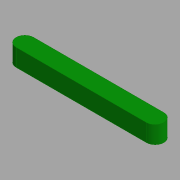
# Autodesk Inventor part: LED green
Saved by Autodesk Inventor 2014 SP2 (Build 180246200, 246)
## iProperties
Created: 2016-01-21
Part Number: LED green
Material: ABS plast
Document SubType Name: Modeling
Designer: Mervart
Mass: 0.0702602 g
Surface Area: 1.3885 cm^2
Volume: 0.0662832 cm^3
Density: 1.06 g/cm^3
Appearance: Hladká – bílá
LastSaveDate: 21.09.2010
Hmotnost: 0
Author: Mervart
Autodesk Inventor part; units mm, degrees
ref_plane "YZ Plane" through (0, 0, 0) normal (1, 0, 0) x (0, 1, 0)
ref_plane "XZ Plane" through (0, 0, 0) normal (0, 1, 0) x (-1, 0, 0)
ref_plane "XY Plane" through (0, 0, 0) normal (0, 0, 1) x (1, 0, 0)
sketch "Náčrt4" plane through (0, 0, 0) normal (0, 0, 1) x (1, 0, 0)
  line L0 (-23.962, 1.2647) -> (-8.962, 1.2647) construction
  line L1 (-8.962, -0.7353) -> (-23.962, -0.7353) construction
  line L2 (-41.962, 1.2647) -> (-26.962, 1.2647) construction
  line L3 (-26.962, -0.7353) -> (-41.962, -0.7353) construction
  line L4 (-59.962, 1.2647) -> (-44.962, 1.2647) construction
  line L5 (-44.962, -0.7353) -> (-59.962, -0.7353) construction
  line L6 (-59.962, 14.7647) -> (-0.822, 14.7647) construction
  arc A0 (-59.962, 14.7647) -> (-69.262, 5.4647) centre (-59.962, 5.4647) ccw construction
  line L7 (-69.262, -84.5353) -> (-69.262, 5.4647) construction
  arc A1 (-69.262, -84.5353) -> (-59.962, -93.8353) centre (-59.962, -84.5353) ccw construction
  line L8 (2.038, -93.8353) -> (-59.962, -93.8353) construction
  line L9 (2.038, -93.8353) -> (2.038, 0.4647) construction
  line L10 (2.038, 0.4647) -> (-0.822, 14.7647) construction
  line L11 (-60.962, -18.7353) -> (-60.962, -4.7353) construction
  line L12 (-59.462, -3.2353) -> (-45.462, -3.2353) construction
  line L13 (-43.962, -4.7353) -> (-43.962, -18.7353) construction
  line L14 (-45.462, -20.2353) -> (-59.462, -20.2353) construction
  circle A2 centre (-34.452, 10.9647) radius 0.3 construction
  circle A3 centre (-30.952, 7.4647) radius 0.3 construction
  circle A4 centre (-34.452, 3.9647) radius 0.3 construction
  circle A5 centre (-37.952, 7.4647) radius 0.3 construction
  circle A6 centre (-34.452, 7.4647) radius 0.3 construction
  circle A7 centre (-36.9269, 9.9395) radius 0.3 construction
  circle A8 centre (-36.9269, 4.9898) radius 0.3 construction
  circle A9 centre (-31.9771, 4.9898) radius 0.3 construction
  circle A10 centre (-31.9771, 9.9395) radius 0.3 construction
  line L15 (-59.962, 1.2647) -> (-44.962, 1.2647)
  line L16 (-44.962, -0.7353) -> (-59.962, -0.7353)
  line L17 (-29.7605, -84.0301) -> (-30.334, -84.8493) projected
  arc A11 (-30.334, -84.8493) -> (-38.5901, -84.8493) centre (-34.462, -90.7447) ccw projected
  line L18 (-38.5901, -84.8493) -> (-39.1636, -84.0301) projected
  arc A12 (-29.7605, -84.0301) -> (-39.1636, -84.0301) centre (-34.462, -90.7447) ccw projected
  circle A13 centre (-34.462, -90.7447) radius 0.9 projected
  line L19 (-31.9385, -86.548) -> (-32.512, -87.3672) projected
  arc A14 (-32.512, -87.3672) -> (-36.412, -87.3672) centre (-34.462, -90.7447) ccw projected
  line L20 (-36.412, -87.3672) -> (-36.9856, -86.548) projected
  arc A15 (-31.9385, -86.548) -> (-36.9856, -86.548) centre (-34.462, -90.7447) ccw projected
  arc A16 (-27.8677, -81.3269) -> (-41.0564, -81.3269) centre (-34.462, -90.7447) ccw projected
  line L21 (-27.8677, -81.3269) -> (-28.4412, -82.1461) projected
  arc A17 (-28.4412, -82.1461) -> (-40.4829, -82.1461) centre (-34.462, -90.7447) ccw projected
  line L22 (-40.4829, -82.1461) -> (-41.0564, -81.3269) projected
  line L23 (-24.962, -72.7353) -> (-24.962, -58.7353) projected
  arc A18 (-23.462, -57.2353) -> (-24.962, -58.7353) centre (-23.462, -58.7353) ccw projected
  line L24 (-23.462, -57.2353) -> (-9.462, -57.2353) projected
  arc A19 (-7.962, -58.7353) -> (-9.462, -57.2353) centre (-9.462, -58.7353) ccw projected
  line L25 (-7.962, -58.7353) -> (-7.962, -72.7353) projected
  arc A20 (-9.462, -74.2353) -> (-7.962, -72.7353) centre (-9.462, -72.7353) ccw projected
  line L26 (-9.462, -74.2353) -> (-23.462, -74.2353) projected
  arc A21 (-24.962, -72.7353) -> (-23.462, -74.2353) centre (-23.462, -72.7353) ccw projected
  line L27 (-42.962, -72.7353) -> (-42.962, -58.7353) projected
  arc A22 (-41.462, -57.2353) -> (-42.962, -58.7353) centre (-41.462, -58.7353) ccw projected
  line L28 (-41.462, -57.2353) -> (-27.462, -57.2353) projected
  arc A23 (-25.962, -58.7353) -> (-27.462, -57.2353) centre (-27.462, -58.7353) ccw projected
  line L29 (-25.962, -58.7353) -> (-25.962, -72.7353) projected
  arc A24 (-27.462, -74.2353) -> (-25.962, -72.7353) centre (-27.462, -72.7353) ccw projected
  line L30 (-27.462, -74.2353) -> (-41.462, -74.2353) projected
  arc A25 (-42.962, -72.7353) -> (-41.462, -74.2353) centre (-41.462, -72.7353) ccw projected
  line L31 (-60.962, -72.7353) -> (-60.962, -58.7353) projected
  arc A26 (-59.462, -57.2353) -> (-60.962, -58.7353) centre (-59.462, -58.7353) ccw projected
  line L32 (-59.462, -57.2353) -> (-45.462, -57.2353) projected
  arc A27 (-43.962, -58.7353) -> (-45.462, -57.2353) centre (-45.462, -58.7353) ccw projected
  line L33 (-43.962, -58.7353) -> (-43.962, -72.7353) projected
  arc A28 (-45.462, -74.2353) -> (-43.962, -72.7353) centre (-45.462, -72.7353) ccw projected
  line L34 (-45.462, -74.2353) -> (-59.462, -74.2353) projected
  arc A29 (-60.962, -72.7353) -> (-59.462, -74.2353) centre (-59.462, -72.7353) ccw projected
  line L35 (-24.962, -54.7353) -> (-24.962, -40.7353) projected
  arc A30 (-23.462, -39.2353) -> (-24.962, -40.7353) centre (-23.462, -40.7353) ccw projected
  line L36 (-23.462, -39.2353) -> (-9.462, -39.2353) projected
  arc A31 (-7.962, -40.7353) -> (-9.462, -39.2353) centre (-9.462, -40.7353) ccw projected
  line L37 (-7.962, -40.7353) -> (-7.962, -54.7353) projected
  arc A32 (-9.462, -56.2353) -> (-7.962, -54.7353) centre (-9.462, -54.7353) ccw projected
  line L38 (-9.462, -56.2353) -> (-23.462, -56.2353) projected
  arc A33 (-24.962, -54.7353) -> (-23.462, -56.2353) centre (-23.462, -54.7353) ccw projected
  line L39 (-42.962, -54.7353) -> (-42.962, -40.7353) projected
  arc A34 (-41.462, -39.2353) -> (-42.962, -40.7353) centre (-41.462, -40.7353) ccw projected
  line L40 (-41.462, -39.2353) -> (-27.462, -39.2353) projected
  arc A35 (-25.962, -40.7353) -> (-27.462, -39.2353) centre (-27.462, -40.7353) ccw projected
  line L41 (-25.962, -40.7353) -> (-25.962, -54.7353) projected
  arc A36 (-27.462, -56.2353) -> (-25.962, -54.7353) centre (-27.462, -54.7353) ccw projected
  line L42 (-27.462, -56.2353) -> (-41.462, -56.2353) projected
  arc A37 (-42.962, -54.7353) -> (-41.462, -56.2353) centre (-41.462, -54.7353) ccw projected
  line L43 (-60.962, -54.7353) -> (-60.962, -40.7353) projected
  arc A38 (-59.462, -39.2353) -> (-60.962, -40.7353) centre (-59.462, -40.7353) ccw projected
  line L44 (-59.462, -39.2353) -> (-45.462, -39.2353) projected
  arc A39 (-43.962, -40.7353) -> (-45.462, -39.2353) centre (-45.462, -40.7353) ccw projected
  line L45 (-43.962, -40.7353) -> (-43.962, -54.7353) projected
  arc A40 (-45.462, -56.2353) -> (-43.962, -54.7353) centre (-45.462, -54.7353) ccw projected
  line L46 (-45.462, -56.2353) -> (-59.462, -56.2353) projected
  arc A41 (-60.962, -54.7353) -> (-59.462, -56.2353) centre (-59.462, -54.7353) ccw projected
  line L47 (-24.962, -36.7353) -> (-24.962, -22.7353) projected
  arc A42 (-23.462, -21.2353) -> (-24.962, -22.7353) centre (-23.462, -22.7353) ccw projected
  line L48 (-23.462, -21.2353) -> (-9.462, -21.2353) projected
  arc A43 (-7.962, -22.7353) -> (-9.462, -21.2353) centre (-9.462, -22.7353) ccw projected
  line L49 (-7.962, -22.7353) -> (-7.962, -36.7353) projected
  arc A44 (-9.462, -38.2353) -> (-7.962, -36.7353) centre (-9.462, -36.7353) ccw projected
  line L50 (-9.462, -38.2353) -> (-23.462, -38.2353) projected
  arc A45 (-24.962, -36.7353) -> (-23.462, -38.2353) centre (-23.462, -36.7353) ccw projected
  line L51 (-42.962, -36.7353) -> (-42.962, -22.7353) projected
  arc A46 (-41.462, -21.2353) -> (-42.962, -22.7353) centre (-41.462, -22.7353) ccw projected
  line L52 (-41.462, -21.2353) -> (-27.462, -21.2353) projected
  arc A47 (-25.962, -22.7353) -> (-27.462, -21.2353) centre (-27.462, -22.7353) ccw projected
  line L53 (-25.962, -22.7353) -> (-25.962, -36.7353) projected
  arc A48 (-27.462, -38.2353) -> (-25.962, -36.7353) centre (-27.462, -36.7353) ccw projected
  line L54 (-27.462, -38.2353) -> (-41.462, -38.2353) projected
  arc A49 (-42.962, -36.7353) -> (-41.462, -38.2353) centre (-41.462, -36.7353) ccw projected
  line L55 (-60.962, -36.7353) -> (-60.962, -22.7353) projected
  arc A50 (-59.462, -21.2353) -> (-60.962, -22.7353) centre (-59.462, -22.7353) ccw projected
  line L56 (-59.462, -21.2353) -> (-45.462, -21.2353) projected
  arc A51 (-43.962, -22.7353) -> (-45.462, -21.2353) centre (-45.462, -22.7353) ccw projected
  line L57 (-43.962, -22.7353) -> (-43.962, -36.7353) projected
  arc A52 (-45.462, -38.2353) -> (-43.962, -36.7353) centre (-45.462, -36.7353) ccw projected
  line L58 (-45.462, -38.2353) -> (-59.462, -38.2353) projected
  arc A53 (-60.962, -36.7353) -> (-59.462, -38.2353) centre (-59.462, -36.7353) ccw projected
  line L59 (-24.962, -18.7353) -> (-24.962, -4.7353) projected
  arc A54 (-23.462, -3.2353) -> (-24.962, -4.7353) centre (-23.462, -4.7353) ccw projected
  line L60 (-23.462, -3.2353) -> (-9.462, -3.2353) projected
  arc A55 (-7.962, -4.7353) -> (-9.462, -3.2353) centre (-9.462, -4.7353) ccw projected
  line L61 (-7.962, -4.7353) -> (-7.962, -18.7353) projected
  arc A56 (-9.462, -20.2353) -> (-7.962, -18.7353) centre (-9.462, -18.7353) ccw projected
  line L62 (-9.462, -20.2353) -> (-23.462, -20.2353) projected
  arc A57 (-24.962, -18.7353) -> (-23.462, -20.2353) centre (-23.462, -18.7353) ccw projected
  line L63 (-42.962, -18.7353) -> (-42.962, -4.7353) projected
  arc A58 (-41.462, -3.2353) -> (-42.962, -4.7353) centre (-41.462, -4.7353) ccw projected
  line L64 (-41.462, -3.2353) -> (-27.462, -3.2353) projected
  arc A59 (-25.962, -4.7353) -> (-27.462, -3.2353) centre (-27.462, -4.7353) ccw projected
  line L65 (-25.962, -4.7353) -> (-25.962, -18.7353) projected
  arc A60 (-27.462, -20.2353) -> (-25.962, -18.7353) centre (-27.462, -18.7353) ccw projected
  line L66 (-27.462, -20.2353) -> (-41.462, -20.2353) projected
  arc A61 (-42.962, -18.7353) -> (-41.462, -20.2353) centre (-41.462, -18.7353) ccw projected
  arc A62 (-23.962, 1.2647) -> (-23.962, -0.7353) centre (-23.962, 0.2647) ccw projected
  arc A63 (-8.962, -0.7353) -> (-8.962, 1.2647) centre (-8.962, 0.2647) ccw projected
  arc A64 (-41.962, 1.2647) -> (-41.962, -0.7353) centre (-41.962, 0.2647) ccw projected
  arc A65 (-26.962, -0.7353) -> (-26.962, 1.2647) centre (-26.962, 0.2647) ccw projected
  arc A66 (-59.962, 1.2647) -> (-59.962, -0.7353) centre (-59.962, 0.2647) ccw projected
  arc A67 (-44.962, -0.7353) -> (-44.962, 1.2647) centre (-44.962, 0.2647) ccw projected
  arc A68 (-59.462, -3.2353) -> (-60.962, -4.7353) centre (-59.462, -4.7353) ccw projected
  arc A69 (-43.962, -4.7353) -> (-45.462, -3.2353) centre (-45.462, -4.7353) ccw projected
  arc A70 (-45.462, -20.2353) -> (-43.962, -18.7353) centre (-45.462, -18.7353) ccw projected
  arc A71 (-60.962, -18.7353) -> (-59.462, -20.2353) centre (-59.462, -18.7353) ccw projected
  point P0 (0, 0)
  point P1 (-43.962, 0.2647)
  constraints: 5 point on circle, 4 end point, 1 horizontal, 1 parallel
extrude "Vysunutí1" add sketch "Náčrt4" against normal blind 2 contours L15 A67 L16 A66
